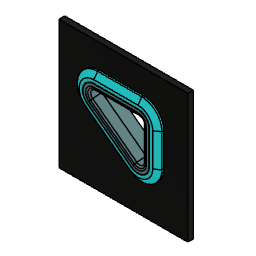
Треугольная гильза v3 (Autodesk Fusion 360 design; units mm, degrees)
Autodesk Fusion 360 part; units mm, degrees
sketch "Sketch1" plane through (0, 0, 0) normal (0, 1, 0) x (1, 0, 0)
  line L0 (-50, -20) -> (20, -20)
  line L1 (20, -20) -> (20, 50)
  line L2 (20, 50) -> (-50, 50)
  line L3 (-50, 50) -> (-50, -20)
  dimension "d1" = 70
  dimension "d2" = 70
  constraint horizontal L0
  constraint vertical L1
  constraint horizontal L2
  constraint vertical L3
  measures "d1" distance of L0.start L0.end
  measures "d2" distance of L0.start L2.end
extrude "Extrude1" add sketch "Sketch1" along normal blind 3 makes body 1
sketch "Sketch2" plane through (0, 0, 0) normal (0, -1, 0) x (1, 0, 0)
  line L0 (-50, 20) -> (-50, -50)
  line L1 (-50, -50) -> (20, -50)
  line L2 (20, -50) -> (20, 20)
  line L3 (20, 20) -> (-50, 20)
  line L4 (-40, 0) -> (0, 0)
  line L5 (0, 0) -> (0, -30)
  line L6 (0, -30) -> (-40, 0)
  circle A0 centre (-28, -4) radius 4
  circle A1 centre (-4, -4) radius 4
  circle A2 centre (-4, -22) radius 4
  dimension "d5" = 40
  dimension "d6" = 30
  dimension "d9" = 8
  constraint horizontal L4
  constraint perpendicular L4 L5
  constraint coincident L4.end L5.start
  constraint equal A0 A1
  constraint equal A1 A2
  constraint tangent L4 A0
  constraint tangent L6 A0
  constraint tangent L4 A1
  constraint tangent L5 A1
  constraint tangent L5 A2
  constraint tangent L6 A2
  measures "d5" distance of L4.start L4.end
  measures "d6" distance of L4.end L5.end
  measures "d9" diameter of A0
extrude "Extrude2" add sketch "Sketch2" against normal blind 8 separate body contours L4 L5 L6 A0 A1 A2 | A0 | A1 | A2 makes body 2
extrude "Extrude3" add 1 faces at (-13.6, 0, -10.8) along direction (0, -1, 0) blind 1.6 on bodies 2 bodies 2
sketch "Sketch3" plane through (0, -1.6, 0) normal (0, -1, 0) x (1, 0, 0)
  arc A0 (-28, 0) -> (-30.4, -7.2) centre (-28, -4) ccw
  line L0 (-30.4, -7.2) -> (-6.4, -25.2)
  arc A1 (-6.4, -25.2) -> (0, -22) centre (-4, -22) ccw
  line L1 (0, -22) -> (0, -4)
  arc A2 (0, -4) -> (-4, 0) centre (-4, -4) ccw
  line L2 (-4, 0) -> (-28, 0)
  line L3 (-4, 2) -> (-28, 2)
  arc A3 (-28, 2) -> (-31.6001, -8.8) centre (-28, -4) ccw
  line L4 (-31.6001, -8.8) -> (-7.6, -26.8)
  arc A4 (-7.6, -26.8) -> (2, -22) centre (-4, -22) ccw
  line L5 (2, -22) -> (2, -4)
  arc A5 (2, -4) -> (-4, 2) centre (-4, -4) ccw
  dimension "d12" = 2
extrude "Extrude4" add sketch "Sketch3" along normal blind 1.5 contours A0 L0 A1 L1 A2 L2 | L3 A3 L4 A4 L5 A5 bodies 2
sketch "Sketch4" plane through (0, -1.6, 0) normal (0, 1, 0) x (-1, 0, 0)
  arc A0 (4, 2) -> (-2, -4) centre (4, -4) ccw
  line L0 (-2, -4) -> (-2, -22)
  arc A1 (-2, -22) -> (7.6, -26.8) centre (4, -22) ccw
  line L1 (7.6, -26.8) -> (31.6001, -8.8)
  arc A2 (31.6001, -8.8) -> (28, 2) centre (28, -4) ccw
  line L2 (28, 2) -> (4, 2)
  line L3 (30.4, -7.2) -> (6.4, -25.2)
  arc A3 (0, -22) -> (6.4, -25.2) centre (4, -22) ccw
  line L4 (0, -22) -> (0, -4)
  arc A4 (4, 0) -> (0, -4) centre (4, -4) ccw
  line L5 (4, 0) -> (28, 0)
  arc A5 (30.4, -7.2) -> (28, 0) centre (28, -4) ccw
  line L6 (4, 0.2) -> (28, 0.2)
  arc A6 (30.52, -7.36) -> (28, 0.2) centre (28, -4) ccw
  line L7 (30.52, -7.36) -> (6.52, -25.36)
  arc A7 (-0.2, -22) -> (6.52, -25.36) centre (4, -22) ccw
  line L8 (-0.2, -22) -> (-0.2, -4)
  arc A8 (4, 0.2) -> (-0.2, -4) centre (4, -4) ccw
  arc A9 (4, 7) -> (-7, -4) centre (4, -4) ccw
  line L9 (-7, -4) -> (-7, -22)
  arc A10 (-7, -22) -> (10.6, -30.8) centre (4, -22) ccw
  line L10 (10.6, -30.8) -> (34.6001, -12.7999)
  arc A11 (34.6001, -12.7999) -> (28, 7) centre (28, -4) ccw
  line L11 (28, 7) -> (4, 7)
  dimension "d15" = 0.2
  dimension "d16" = 5
extrude "Extrude5" add sketch "Sketch4" along normal up to surface (1.5 mm away) separate body contours A0 L0 A1 L1 A2 L2 | A9 L9 A10 L10 A11 L11 makes body 3
sketch "Sketch5" plane through (0, -1.6, 0) normal (0, -1, 0) x (1, 0, 0)
  arc A0 (-28, 0.2) -> (-30.52, -7.36) centre (-28, -4) ccw
  line L0 (-28, 0.2) -> (-4, 0.2)
  arc A1 (0.2, -4) -> (-4, 0.2) centre (-4, -4) ccw
  line L1 (0.2, -4) -> (0.2, -22)
  arc A2 (-6.52, -25.36) -> (0.2, -22) centre (-4, -22) ccw
  line L2 (-6.52, -25.36) -> (-30.52, -7.36)
  line L3 (-4, 7) -> (-28, 7)
  arc A3 (-28, 7) -> (-34.6001, -12.7999) centre (-28, -4) ccw
  line L4 (-34.6001, -12.7999) -> (-10.6, -30.8)
  arc A4 (-10.6, -30.8) -> (7, -22) centre (-4, -22) ccw
  line L5 (7, -22) -> (7, -4)
  arc A5 (7, -4) -> (-4, 7) centre (-4, -4) ccw
  arc A6 (2, -4) -> (-4, 2) centre (-4, -4) ccw
  line L6 (-4, 2) -> (-28, 2)
  arc A7 (-28, 2) -> (-31.6001, -8.8) centre (-28, -4) ccw
  line L7 (-31.6001, -8.8) -> (-7.6, -26.8)
  arc A8 (-7.6, -26.8) -> (2, -22) centre (-4, -22) ccw
  line L8 (2, -22) -> (2, -4)
  line L9 (-4, 2.2) -> (-28, 2.2)
  arc A9 (-28, 2.2) -> (-31.7201, -8.96) centre (-28, -4) ccw
  line L10 (-31.7201, -8.96) -> (-7.72, -26.96)
  arc A10 (-7.72, -26.96) -> (2.2, -22) centre (-4, -22) ccw
  line L11 (2.2, -22) -> (2.2, -4)
  arc A11 (2.2, -4) -> (-4, 2.2) centre (-4, -4) ccw
  dimension "d19" = 0.2
extrude "Extrude6" add sketch "Sketch5" along normal up to surface (1.5 mm away) contours L3 A3 L4 A4 L5 A5 bodies 3
chamfer "Chamfer1" distance 2 distance2 3 6 edges at (0.9193, -3.1, -31.8387) (-22.6, -3.1, -21.8) (-38.4355, -3.1, -0.5215) (-16, -3.1, 7) (3.7782, -3.1, 3.7782) (7, -3.1, -13) measured on face at (-9.7034, -1.6, -31.4059) measured on face at (-26.6001, -2.1, -18.8) measured on face at (-35.4291, -1.6, -12.1122) measured on face at (-12, -2.1, 7) measured on face at (-2.9544, -1.6, 6.9502) measured on face at (7, -1.1, -16) on bodies 3
sketch "Sketch6" plane through (0, 8, 0) normal (0, 1, 0) x (-1, 0, 0)
  arc A0 (30.4, -7.2) -> (28, 0) centre (28, -4) ccw
  line L0 (28, 0) -> (4, 0)
  arc A1 (4, 0) -> (0, -4) centre (4, -4) ccw
  line L1 (0, -4) -> (0, -22)
  arc A2 (0, -22) -> (6.4, -25.2) centre (4, -22) ccw
  line L2 (6.4, -25.2) -> (30.4, -7.2)
  arc A3 (3, -22) -> (4.6, -22.8) centre (4, -22) ccw
  line L3 (4.6, -22.8) -> (28.6, -4.8)
  arc A4 (28.6, -4.8) -> (28, -3) centre (28, -4) ccw
  line L4 (28, -3) -> (4, -3)
  arc A5 (4, -3) -> (3, -4) centre (4, -4) ccw
  line L5 (3, -4) -> (3, -22)
  dimension "d24" = -3
extrude "Extrude7" cut sketch "Sketch6" against normal up to surface (11.1 mm away) contours A3 L3 A4 L4 A5 L5 bodies 2
chamfer "Chamfer2" distance 2 distance2 5 6 edges at (-16.6, -3.1, -13.8) (-28.9487, -3.1, -3.6838) (-16, -3.1, -3) (-3.2929, -3.1, -3.2929) (-3, -3.1, -13) (-3.5528, -3.1, -22.8944) measured on face at (-22.6, -3.1, -13.4666) measured on face at (-22.6, -3.1, -13.4666) measured on face at (-22.6, -3.1, -13.4666) measured on face at (-22.6, -3.1, -13.4666) measured on face at (-22.6, -3.1, -13.4666) measured on face at (-22.6, -3.1, -13.4666) on bodies 2
ref_plane "WorkPlane1" through (-15, 3.1, -15) normal (0, 1, 0) x (0, 0, 1)
sketch "Sketch7" plane through (0.8764, 3.1, -2.488) normal (0, 1, 0) x (1, 0, 0)
  line L0 (-4.8764, 0.512) -> (-28.8764, 0.512)
  arc A0 (-29.4764, 2.312) -> (-28.8764, 0.512) centre (-28.8764, 1.512) ccw
  line L1 (-29.4764, 2.312) -> (-5.4764, 20.312)
  arc A1 (-3.8764, 19.512) -> (-5.4764, 20.312) centre (-4.8764, 19.512) ccw
  line L2 (-3.8764, 19.512) -> (-3.8764, 1.512)
  arc A2 (-4.8764, 0.512) -> (-3.8764, 1.512) centre (-4.8764, 1.512) ccw
  arc A3 (-31.2764, 4.712) -> (-28.8764, -2.488) centre (-28.8764, 1.512) ccw
  line L3 (-28.8764, -2.488) -> (-4.8764, -2.488)
  arc A4 (-4.8764, -2.488) -> (-0.8764, 1.512) centre (-4.8764, 1.512) ccw
  line L4 (-0.8764, 1.512) -> (-0.8764, 19.512)
  arc A5 (-0.8764, 19.512) -> (-7.2764, 22.712) centre (-4.8764, 19.512) ccw
  line L5 (-7.2764, 22.712) -> (-31.2764, 4.712)
ref_plane "WorkPlane2" through (0, 0, -10) normal (0, 0, 1) x (1, 0, 0)
sketch "Sketch8" plane through (0, 0, -10) normal (0, 0, 1) x (1, 0, 0)
  line L0 (0, 4.3) -> (-1.2, 4.3)
  line L1 (-1.2, 4.3) -> (-1.2, 3.1)
  line L2 (-1.2, 3.1) -> (0, 3.1)
  line L3 (0, 3.1) -> (0, 4.3)
  point P0 (0, 3.1)
  dimension "d31" = 1.2
  dimension "d32" = 1.2
  constraint horizontal L0
  constraint vertical L1
  constraint horizontal L2
  constraint vertical L3
  constraint coincident P0 L2.end
  measures "d31" distance of L0.start L0.end
  measures "d32" distance of L0.start P0
sweep "Sweep1" cut profiles "Sketch8" path "Sketch7" along L5 A3 L3 A4 L4 A5 section 1 bodies 2
chamfer "Chamfer3" distance 1.5 distance2 1.2 6 edges at (-2.2112, 4.3, -25.5777) (-18.4, 4.3, -16.2) (-31.7947, 4.3, -2.7351) (-16, 4.3, 0) (-1.1716, 4.3, -1.1716) (0, 4.3, -13) measured on face at (-0.0048, 5.5333, -22.1967) measured on face at (-14.4, 6.7667, -19.2) measured on face at (-30.5538, 6.7667, -7.0786) measured on face at (-12, 5.5333, 0) measured on face at (-0.0045, 6.7667, -3.8097) measured on face at (0, 6.7667, -16) on bodies 2
sketch "Sketch9" plane through (0, 3.1, 0) normal (0, 1, 0) x (-1, 0, 0)
  line L0 (0, -4) -> (0, -22)
  arc A0 (0, -22) -> (6.4, -25.2) centre (4, -22) ccw
  line L1 (6.4, -25.2) -> (30.4, -7.2)
  arc A1 (30.4, -7.2) -> (28, 0) centre (28, -4) ccw
  line L2 (28, 0) -> (4, 0)
  arc A2 (4, 0) -> (0, -4) centre (4, -4) ccw
  arc A3 (1.2, -22) -> (5.68, -24.24) centre (4, -22) ccw
  line L3 (1.2, -22) -> (1.2, -4)
  arc A4 (4, -1.2) -> (1.2, -4) centre (4, -4) ccw
  line L4 (4, -1.2) -> (28, -1.2)
  arc A5 (29.68, -6.24) -> (28, -1.2) centre (28, -4) ccw
  line L5 (29.68, -6.24) -> (5.68, -24.24)
  line L6 (4, -3) -> (28, -3)
  arc A6 (28.6, -4.8) -> (28, -3) centre (28, -4) ccw
  line L7 (28.6, -4.8) -> (4.6, -22.8)
  arc A7 (3, -22) -> (4.6, -22.8) centre (4, -22) ccw
  line L8 (3, -22) -> (3, -4)
  arc A8 (4, -3) -> (3, -4) centre (4, -4) ccw
  arc A9 (30.4, -7.2) -> (28, 0) centre (28, -4) ccw construction
  line L9 (28, 0) -> (4, 0) construction
  arc A10 (4, 0) -> (0, -4) centre (4, -4) ccw construction
  line L10 (0, -4) -> (0, -22) construction
  arc A11 (0, -22) -> (6.4, -25.2) centre (4, -22) ccw construction
  line L11 (6.4, -25.2) -> (30.4, -7.2) construction
  arc A12 (4, 2) -> (-2, -4) centre (4, -4) ccw
  line L12 (-2, -4) -> (-2, -22)
  arc A13 (-2, -22) -> (7.6, -26.8) centre (4, -22) ccw
  line L13 (7.6, -26.8) -> (31.6001, -8.8)
  arc A14 (31.6001, -8.8) -> (28, 2) centre (28, -4) ccw
  line L14 (28, 2) -> (4, 2)
  dimension "d41" = 2
extrude "Extrude8" add sketch "Sketch9" along normal blind 2 separate body contours L0 A0 L1 A1 L2 A2 | A3 L3 A4 L4 A5 L5 | A12 L12 A13 L13 A14 L14 makes body 4
combine "Combine1" operation cut target body 4 tool bodies 2 keep tools
combine "Combine2" operation cut target body 1 tool bodies 2 keep tools makes body 5 at (-12.704, 0, -10.352)
sketch "Sketch10" plane through (0, 3.1, 0) normal (0, -1, 0) x (1, 0, 0)
  arc A0 (-1.2, -4) -> (-4, -1.2) centre (-4, -4) ccw
  line L0 (-1.2, -4) -> (-1.2, -22)
  arc A1 (-5.68, -24.24) -> (-1.2, -22) centre (-4, -22) ccw
  line L1 (-5.68, -24.24) -> (-29.68, -6.24)
  arc A2 (-28, -1.2) -> (-29.68, -6.24) centre (-28, -4) ccw
  line L2 (-28, -1.2) -> (-4, -1.2)
  line L3 (-4, 2) -> (-28, 2)
  arc A3 (-28, 2) -> (-31.6001, -8.8) centre (-28, -4) ccw
  line L4 (-31.6001, -8.8) -> (-7.6, -26.8)
  arc A4 (-7.6, -26.8) -> (2, -22) centre (-4, -22) ccw
  line L5 (2, -22) -> (2, -4)
  arc A5 (2, -4) -> (-4, 2) centre (-4, -4) ccw
  arc A6 (-5.74, -24.32) -> (-1.1, -22) centre (-4, -22) ccw
  line L6 (-1.1, -4) -> (-1.1, -22)
  arc A7 (-1.1, -4) -> (-4, -1.1) centre (-4, -4) ccw
  line L7 (-28, -1.1) -> (-4, -1.1)
  arc A8 (-28, -1.1) -> (-29.74, -6.32) centre (-28, -4) ccw
  line L8 (-5.74, -24.32) -> (-29.74, -6.32)
  line L9 (2, -13.15) -> (0.9777, -13.15)
  line L10 (0.9777, -13.15) -> (-0.1668, -12.4046)
  line L11 (-0.1668, -12.4046) -> (-1.1, -12.4046)
  line L12 (2, -12.85) -> (1.0668, -12.85)
  line L13 (1.0668, -12.85) -> (-0.0777, -12.1046)
  line L14 (-0.0777, -12.1046) -> (-1.1, -12.1046)
  line L15 (2, -13) -> (4, -13) construction
  dimension "d44" = -0.1
  dimension "d47" = 0.3
  dimension "d48" = 0.3
  dimension "d49" = 0.3
  constraint coincident L5 L9.start
  constraint perpendicular L5 L9
  constraint coincident L6 L11.end
  constraint perpendicular L6 L11
  constraint coincident L5 L12.start
  constraint perpendicular L5 L12
  constraint coincident L6 L14.end
  constraint perpendicular L6 L14
  constraint midpoint L5 L15.start
  constraint perpendicular L5 L15
  constraint parallel L10 L13
  constraint equal L9 L14
  measures "d47" distance of L9 L12
  measures "d48" distance of L11 L14
  measures "d49" distance of L10 L13
extrude "Extrude9" cut sketch "Sketch10" against normal up to surface (2 mm away) contours L5 L6 L9 L10 L11 L12 L13 L14 | A6 L6 A7 L7 A8 L8 bodies 4
chamfer "Chamfer4" distance 1 angle 45 6 edges at (-1, -3.1, -13) (-1.8787, -3.1, -1.8787) (-16, -3.1, -1) (-30.846, -3.1, -3.0513) (-17.8, -3.1, -15.4) (-2.6584, -3.1, -24.6833) on bodies 2
chamfer "Chamfer5" distance 0.5 angle 45 6 edges at (-16, -3.1, 0) (-31.7947, -3.1, -2.7351) (-18.4, -3.1, -16.2) (-2.2112, -3.1, -25.5777) (0, -3.1, -13) (-1.1716, -3.1, -1.1716) on bodies 2
hidden bodies 5
equation "d48 = d47"
equation "d49 = d47"
